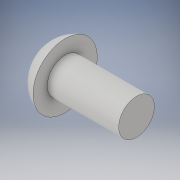
# Autodesk Inventor part: Screw (train)
Saved by Autodesk Inventor 2017 (Build 210142000, 142)
## iProperties
Created: 2017-04-26
Part Number: Screw (train)
Material: Generic
Document SubType Name: Modeling
Designer: 193515
Density: 1 g/cm^3
Appearance: Default
Author: 193515
Autodesk Inventor part; units mm, degrees
ref_plane "YZ Plane" through (0, 0, 0) normal (1, 0, 0) x (0, 1, 0)
ref_plane "XZ Plane" through (0, 0, 0) normal (0, 1, 0) x (-1, 0, 0)
ref_plane "XY Plane" through (0, 0, 0) normal (0, 0, 1) x (1, 0, 0)
sketch "Sketch1" plane through (0, 0, 0) normal (0, 0, 1) x (1, 0, 0)
  line L0 (0, -3.33) -> (-12.7, -3.33)
  line L1 (-12.7, -3.33) -> (-12.7, -0.79)
  line L2 (0, -3.33) -> (0, -6.505)
  line L3 (0, -6.505) -> (-16.51, -6.505)
  arc A0 (-12.7, -0.79) -> (-16.51, -6.505) centre (-11.2646, -5.8744) ccw
  point P0 (0, 0)
  dimension "d0" = 12.7
  dimension "d1" = 2.54
  dimension "d2" = 3.175
  dimension "d3" = 16.51
  dimension "d4" = 5.2832
  constraints: 8 end point, 2 point on circle, 2 vertical, 1 centre point, 1 horizontal, 1 perpendicular
  measures "d0" distance of L0.start L0.end
  measures "d1" distance of L0.end L1.end
  measures "d2" distance of L0.start L2.end
  measures "d3" distance of L2.end L3.end
  measures "d4" radius of A0
revolve "Revolution1" add sketch "Sketch1" angle 360 about axis through (0, -6.505, 0) along (-1, 0, 0)
body "Solid1"
